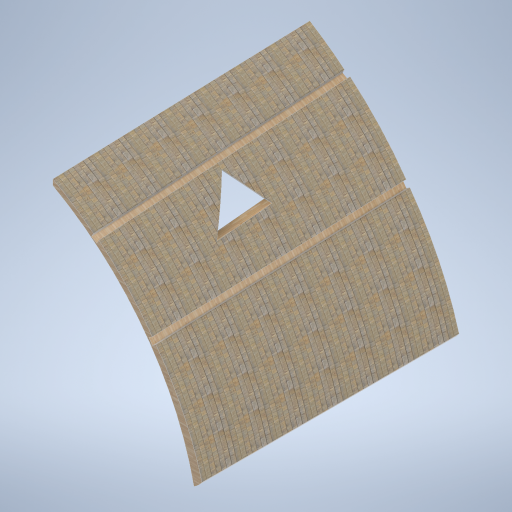
# Autodesk Inventor part: panel_block_03
Saved by Autodesk Inventor 2024.2 (Build 282272000, 272)
## iProperties
Created: 2024-05-21
Part Number: panel_block_03
Material: Wood (Maple)
Document SubType Name: Modeling
Designer: LOSTER_1
Density: 0.67 g/cm^3
Appearance: Natural Maple - Glossy Dark Tint
Author: LOSTER_1
Autodesk Inventor part; units mm, degrees
ref_plane "XZ Plane" through (0, 0, 0) normal (0, 1, 0) x (-1, 0, 0)
sketch "Sketch1" plane through (0, 0, 0) normal (0, 0, 1) x (1, 0, 0)
  arc A0 (4796.3585, -1909.6289) -> (3343.4744, 1121.5056) centre (-3903.1767, -4215.7265) ccw
  line L0 (3236.8192, 1046.7661) -> (3343.5051, 1121.464)
  arc A1 (3228.7635, 1285.3391) -> (1546.1726, 3076.3751) centre (-4110.5601, -3923.7232) ccw
  line L1 (3228.7635, 1285.3391) -> (3122.0787, 1210.6419)
  line L2 (1372.9503, 3176.3452) -> (1308.1705, 3064.1503)
  arc A2 (1372.9503, 3176.3452) -> (93.8576, 4024.2684) centre (-4221.2651, -3873.8147) ccw
  line L3 (1481.3729, 2964.1457) -> (1546.1726, 3076.3751)
  arc A3 (4543.4821, -2147.4888) -> (93.8528, 3844.2289) centre (-4256.4671, -4034.5221) ccw
  line L4 (93.8576, 4024.2684) -> (93.8528, 3844.2289)
  line L5 (1308.1705, 3064.1503) -> (1481.3729, 2964.1457)
  line L6 (3122.0787, 1210.6419) -> (3236.8192, 1046.7661)
  arc A4 (4543.4821, -2147.4888) -> (4796.3585, -1909.6289) centre (4134.8595, -1459.7188) ccw
  point P0 (0, 0)
  dimension "d7" = 800
  constraints: 14 end point, 11 point on circle, 5 centre point, 1 perpendicular
  measures "d7" radius of A4
ref_plane "Work Plane2" through (0, 0, -8101) normal (0, 0, 1) x (1, 0, 0)
ref_plane "Work Plane1" through (0, 0, 0) normal (0, 0, 1) x (1, 0, 0)
sketch "Sketch2" plane through (0, 0, -8101) normal (0, 0, 1) x (1, 0, 0)
  arc A0 (1192.0552, 3508.338) -> (93.8528, 4294.485) centre (-5164.5547, -4211.3454) ccw projected
  arc A1 (3133.8513, 1483.0798) -> (1365.2603, 3408.338) centre (-5051.6105, -4261.3276) ccw projected
  arc A2 (4543.6426, -2147.8414) -> (93.8528, 4114.0508) centre (-5207.4444, -4365.1147) ccw projected
  line L0 (1192.0552, 3508.338) -> (1126.9741, 3395.6142) projected
  line L1 (1365.2603, 3408.338) -> (1300.1792, 3295.6142) projected
  line L2 (1126.9741, 3395.6142) -> (1300.1792, 3295.6142) projected
  line L3 (93.8528, 4294.485) -> (93.8528, 4114.0508) projected
  line L4 (3027.6129, 1408.6909) -> (3133.8513, 1483.0798) projected
  line L5 (3142.3282, 1244.8605) -> (3248.5665, 1319.2494) projected
  line L6 (3027.6129, 1408.6909) -> (3142.3282, 1244.8605) projected
  arc A3 (4803.6655, -1899.2732) -> (3248.5665, 1319.2494) centre (-4832.968, -4570.4704) ccw projected
  arc A4 (4543.6426, -2147.8414) -> (4803.6655, -1899.2732) centre (4135.0016, -1460.0824) ccw projected
  point P0 (0, 0)
loft "Loft1" add profiles "Sketch1", "Sketch2"
ref_plane "Work Plane3" through (2600, 0, 0) normal (1, 0, 0) x (0, 1, 0)
sketch "Sketch3" plane through (2600, 0, 0) normal (1, 0, 0) x (0, 1, 0)
  line L0 (3120.8038, -3828.6818) -> (2179.9067, -2717.5683)
  line L1 (2179.9067, -2717.5683) -> (2281.1646, -4539.693)
  line L2 (2281.1646, -4539.693) -> (3120.8038, -3828.6818)
  point P0 (0, 0)
  constraints: 6 end point, 1 perpendicular
extrude "Extrusion1" cut sketch "Sketch3" against normal through all
body "Solid1"
